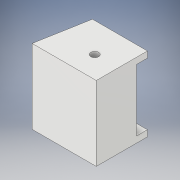
# Autodesk Inventor part: AA016
Saved by Autodesk Inventor 2017 SP1 (Build 210196100, 196)
## iProperties
Created: 2017-09-29
Part Number: AA016
Material: ABS Plastic
Document SubType Name: Modeling
Designer: Zach
Density: 1.06 g/cm^3
Appearance: CR White
Author: Zach
Autodesk Inventor part; units mm, degrees
ref_plane "YZ Plane" through (0, 0, 0) normal (1, 0, 0) x (0, 1, 0)
ref_plane "XZ Plane" through (0, 0, 0) normal (0, 1, 0) x (-1, 0, 0)
ref_plane "XY Plane" through (0, 0, 0) normal (0, 0, 1) x (1, 0, 0)
sketch "Sketch1" plane through (0, 0, 0) normal (0, 0, 1) x (1, 0, 0)
  line L0 (0, 0) -> (70, 0)
  line L1 (70, 0) -> (70, 77.5)
  line L2 (70, 77.5) -> (0, 77.5)
  line L3 (0, 77.5) -> (0, 0)
  dimension "d0" = 70
  dimension "d1" = 77.5
  constraints: 8 end point, 2 parallel, 1 horizontal, 1 perpendicular
  measures "d0" distance of L2.end L1.end
  measures "d1" distance of L1.end L0.end
extrude "Extrusion1" add sketch "Sketch1" along normal blind 70
sketch "Sketch3" plane through (0, 0, 70) normal (0, 0, 1) x (1, 0, 0)
  line L0 (0, 0) -> (70, 0) projected
  line L1 (70, 77.5) -> (0, 77.5) projected
  line L2 (70, 0) -> (35, 0)
  line L3 (35, 0) -> (35, 77.5)
  line L4 (35, 77.5) -> (70, 77.5)
  line L5 (70, 77.5) -> (70, 0)
  constraints: 8 end point, 2 parallel, 1 horizontal, 1 midpoint, 1 perpendicular
extrude "Extrusion3" cut sketch "Sketch3" against normal through all
sketch "Sketch4" plane through (0, 77.5, 70) normal (0, 1, 0) x (1, 0, 0)
  line L0 (0, 70) -> (0, 0) projected
  line L1 (0, 0) -> (-12.5, 0)
  line L2 (35, 70) -> (0, 70) projected
  arc A0 (-12.5, 0) -> (0, 70) centre (-1137.8005, 237.0626) ccw
  line L3 (-12.5, -10) -> (35, -10) construction
  dimension "d9" = 1150
  dimension "d54" = 47.5
  dimension "d55" = 10
  constraints: 4 end point, 2 horizontal, 2 point on circle, 2 vertical alignment, 1 centre point
  measures "d9" radius of A0
  measures "d54" distance of L3.start L3.end
  measures "d55" distance between parallel lines of L1 L3
extrude "Extrusion4" add sketch "Sketch4" against normal blind 77.5
sketch "Sketch5" plane through (35, 0, 70) normal (1, 0, 0) x (0, 0, -1)
  line L0 (0, 77.5) -> (0, 86.25)
  line L1 (0, 0) -> (0, -8.75)
  line L2 (0, 0) -> (0, 77.5) projected
  line L3 (70, 77.5) -> (70, 0) projected
  arc A0 (0, 86.25) -> (70, 77.5) centre (177.5728, 1222.4577) ccw
  arc A1 (70, 0) -> (0, -8.75) centre (177.5728, -1144.9577) ccw
  line L4 (0, 77.5) -> (70, 77.5) projected
  line L5 (70, 0) -> (0, 0) projected
  line L6 (-10, 86.25) -> (-10, -8.75) construction
  point P0 (-10, 38.75)
  point P1 (0, 38.75)
  dimension "d14" = 1150
  dimension "d15" = 1150
  dimension "d52" = 10
  dimension "d53" = 95
  constraints: 6 end point, 4 point on circle, 3 horizontal alignment, 3 vertical, 2 centre point, 2 midpoint
  measures "d14" radius of A0
  measures "d15" radius of A1
  measures "d52" distance between parallel lines of L2 L6
  measures "d53" distance of L6.start L6.end
extrude "Extrusion5" add sketch "Sketch5" against normal blind 55 contours L0 A0 L4 | L5 A1 L1
sketch "Sketch6" plane through (-20, 0, 0) normal (0, 1, 0) x (1, 0, 0)
  line L0 (20, 0) -> (0, 0) projected
  line L1 (0, -70) -> (0, 0) projected
  arc A0 (7.5, -70) -> (20, 0) centre (-1117.8005, 167.0626) ccw projected
  line L2 (7.5, -70) -> (0, -70) projected
extrude "Extrusion6" cut sketch "Sketch6" along normal through all both and the other way through all
fillet "Fillet3" radius 19.35 2 edges at (-5.7463, 81.368, 35.3063) (-5.7463, -3.868, 35.3063)
sketch "Sketch8" plane through (0, 0, 70) normal (0, 0, 1) x (1, 0, 0)
  line L0 (35, 86.25) -> (35, -8.75) projected
  line L1 (35, 77.5) -> (35, 0) projected
  circle A0 centre (35, 38.75) radius 35
  point P0 (0, 0)
  dimension "d23" = 70
  constraints: 1 centre point, 1 midpoint
  measures "d23" diameter of A0
extrude "Extrusion7" cut sketch "Sketch8" against normal blind 17.5
sketch "Sketch17" plane through (35, 0, 0) normal (1, 0, 0) x (0, 0, -1)
  line L0 (-5, 13.75) -> (-40, 13.75)
  line L1 (-40, 13.75) -> (-40, 63.75)
  line L2 (-40, 63.75) -> (-5, 63.75)
  line L3 (-5, 63.75) -> (-5, 13.75)
  line L4 (0, 77.5) -> (0, 0) projected
  line L5 (-70, 86.25) -> (-70, 73.75) projected
  arc A0 (-70, 86.25) -> (0, 77.5) centre (107.5728, 1222.4577) ccw projected
  line L6 (-70, 3.75) -> (-70, 73.75) projected
  line L7 (-70, 3.75) -> (-70, -8.75) projected
  arc A1 (0, 0) -> (-70, -8.75) centre (107.5728, -1144.9577) ccw projected
  point P0 (-5, 38.75)
  point P1 (0, 38.75)
  dimension "d62" = 35
  dimension "d63" = 50
  dimension "d77" = 5
  constraints: 8 end point, 2 midpoint, 2 parallel, 1 horizontal, 1 horizontal alignment, 1 perpendicular
  measures "d62" distance of L1.end L2.end
  measures "d63" distance of L0.end L1.end
  measures "d77" distance between parallel lines of L4 L3
extrude "Extrusion15" cut sketch "Sketch17" against normal through all
sketch "Sketch21" plane through (35, 13.75, 5) normal (1, 0, 0) x (0, 0, -1)
  line L0 (-8, 5) -> (0, 5)
  line L1 (0, 5) -> (0, 45)
  line L2 (0, 45) -> (-8, 45)
  line L3 (-8, 45) -> (-8, 5)
  line L4 (0, 0) -> (0, 50) projected
  point P0 (5, -13.75)
  point P1 (-35, 25)
  point P2 (0, 25)
  dimension "d78" = 40
  dimension "d79" = 8
  constraints: 8 end point, 2 midpoint, 2 parallel, 1 horizontal, 1 perpendicular
  measures "d78" distance of L0.end L1.end
  measures "d79" distance of L1.end L2.end
extrude "Extrusion19" cut sketch "Sketch21" against normal blind 30
sketch "Sketch22" plane through (35, 63.75, 40) normal (0, 1, 0) x (1, 0, 0)
  line L0 (0, 35) -> (0, 0) projected
  circle A0 centre (-15, 15) radius 2.5
  line L1 (0, 35) -> (-35.1041, 35) projected
  point P0 (-35, 40)
  dimension "d82" = 5
  dimension "d90" = 20
  dimension "d91" = 15
  constraints: 1 centre point
  measures "d82" diameter of A0
  measures "d90" distance from line of L1 A0.centre
  measures "d91" distance from line of L0 A0.centre
extrude "Extrusion20" cut sketch "Sketch22" against normal through all
sketch "Sketch23" plane through (35, 13.75, 40) normal (1, 0, 0) x (0, 0, -1)
  line L0 (35, 5) -> (27, 5) construction
  line L1 (27, 5) -> (27, 45) construction
  line L2 (27, 45) -> (35, 45) construction
  line L3 (35, 45) -> (35, 50) construction
  line L4 (35, 50) -> (0, 50) construction
  line L5 (0, 50) -> (0, 0) construction
  line L6 (0, 0) -> (35, 0) construction
  line L7 (35, 0) -> (35, 5) construction
  line L8 (35, 50) -> (0, 50) projected
  line L9 (0, 50) -> (35, 50)
  line L10 (35, 50) -> (35, 0)
  line L11 (35, 0) -> (0, 0)
  line L12 (0, 0) -> (0, 50)
  line L13 (34, 1) -> (34, 49)
  line L14 (34, 49) -> (1, 49)
  line L15 (1, 49) -> (1, 1)
  line L16 (1, 1) -> (34, 1)
  point P0 (40, -13.75)
  dimension "d86" = 1
  constraints: 16 end point, 4 parallel, 2 perpendicular, 1 horizontal, 3 other
  measures "d86" distance between parallel lines of L10 L13
extrude "Extrusion21" cut sketch "Sketch23" against normal through all
body "Solid1"
